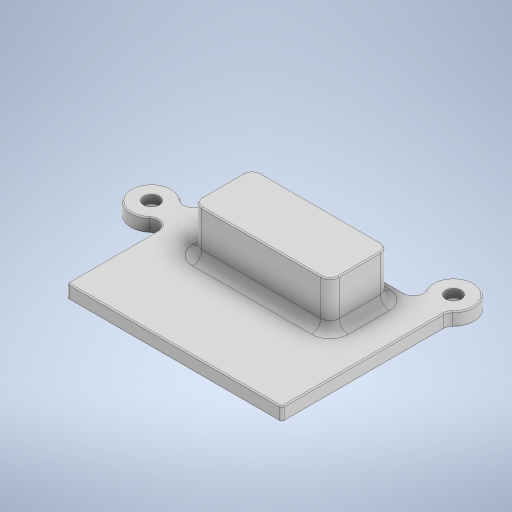
# Autodesk Inventor part: v2breadboardmount
Saved by Autodesk Inventor 2024.2 (Build 282272000, 272)
## iProperties
Created: 2024-01-13
Part Number: v2breadboardmount
Material: Generic
Document SubType Name: Modeling
Designer: Eric
Density: 1 g/cm^3
Appearance: Default
Author: Eric
Autodesk Inventor part; units mm, degrees
ref_plane "YZ Plane" through (0, 0, 0) normal (1, 0, 0) x (0, 1, 0)
ref_plane "XZ Plane" through (0, 0, 0) normal (0, 1, 0) x (-1, 0, 0)
ref_plane "XY Plane" through (0, 0, 0) normal (0, 0, 1) x (1, 0, 0)
sketch "Sketch1" plane through (0, 0, 0) normal (0, 1, 0) x (-1, 0, 0)
  line L0 (23.5, 17.5) -> (-23.5, 17.5)
  line L1 (-23.5, 17.5) -> (-23.5, -17.5)
  line L2 (-23.5, -17.5) -> (23.5, -17.5)
  line L3 (23.5, -17.5) -> (23.5, 17.5)
  line L4 (23.5, 17.5) -> (-23.5, -17.5) construction
  line L5 (-23.5, 17.5) -> (23.5, -17.5) construction
  circle A0 centre (-21, -22.5) radius 1.7
  circle A1 centre (-21, -22.5) radius 4.5
  line L6 (-23.5, -18.7583) -> (-23.5, -17.5)
  line L7 (-18.5, -17.5) -> (-18.5, -18.7583)
  circle A2 centre (29.8, -7.3) radius 1.7
  circle A3 centre (29.8, -7.3) radius 4.5
  line L8 (26.0583, -9.8) -> (23.5, -9.8)
  line L9 (23.5, -4.8) -> (26.0583, -4.8)
  point P0 (0, 0)
  point P1 (-16.8117, -24.1455)
  dimension "d0" = 47
  dimension "d1" = 35
  dimension "d3" = 3.4
  dimension "d4" = 5
  dimension "d5" = 9
  dimension "d17" = 2.5
  dimension "d18" = 5
  dimension "d19" = 50.8
  dimension "d20" = 5
  dimension "d21" = 2.5
  dimension "d22" = 15.2
  constraints: 20 end point, 5 point on circle, 4 centre point, 4 point on line, 3 parallel, 3 perpendicular, 2 coincident, 2 equal radius, 2 midpoint, 1 collinear, 1 horizontal, 1 vertical
  measures "d0" distance of L1.end L2.end
  measures "d1" distance between parallel lines of L0 L2
  measures "d3" diameter of A0
  measures "d4" distance from line of L2 A0.centre
  measures "d5" diameter of A1
  measures "d17" distance from line of L6 A0.centre
  measures "d18" distance between parallel lines of L6 L7
  measures "d19" horizontal distance of A0.centre A2.centre
  measures "d20" distance between parallel lines of L8 L9
  measures "d21" distance from line of L8 A2.centre
  measures "d22" vertical distance of A0.centre A2.centre
extrude "Extrusion1" add sketch "Sketch1" against normal blind 3
sketch "Sketch3" plane through (0, -3, 0) normal (0, 1, 0) x (1, 0, 0)
  circle A0 centre (-29.8, 7.3) radius 1.7 projected
  line L0 (-28.1546, 4.45) -> (-31.4454, 4.45)
  line L1 (-31.4454, 4.45) -> (-33.0909, 7.3)
  line L2 (-33.0909, 7.3) -> (-31.4454, 10.15)
  line L3 (-31.4454, 10.15) -> (-28.1546, 10.15)
  line L4 (-28.1546, 10.15) -> (-26.5091, 7.3)
  line L5 (-26.5091, 7.3) -> (-28.1546, 4.45)
  circle A1 centre (21, 22.5) radius 1.7 projected
  line L6 (21, 19.2091) -> (18.15, 20.8546)
  line L7 (18.15, 20.8546) -> (18.15, 24.1454)
  line L8 (18.15, 24.1454) -> (21, 25.7909)
  line L9 (21, 25.7909) -> (23.85, 24.1454)
  line L10 (23.85, 24.1454) -> (23.85, 20.8546)
  line L11 (23.85, 20.8546) -> (21, 19.2091)
  point P0 (0, 0)
  dimension "d23" = 5.7
  constraints: 24 end point, 2 coincident, 1 horizontal, 1 perpendicular, 1 vertical, 26 other
  measures "d23" distance between parallel lines of L10 L7
extrude "Extrusion3" cut sketch "Sketch3" along normal blind 1 contours A0 | L0 L1 L2 L3 L4 L5 | A1 | L6 L7 L8 L9 L10 L11
sketch "Sketch4" plane through (0, 0, 0) normal (0, 1, 0) x (1, 0, 0)
  line L0 (-15, 14.5) -> (15, 14.5)
  line L1 (15, 14.5) -> (15, 1.5)
  line L2 (15, 1.5) -> (-15, 1.5)
  line L3 (-15, 1.5) -> (-15, 14.5)
  line L4 (18.5, 17.5) -> (-23.5, 17.5) projected
  point P0 (0, 0)
  point P1 (0, 1.5)
  dimension "d26" = 30
  dimension "d27" = 13
  dimension "d28" = 3
  constraints: 8 end point, 2 parallel, 1 horizontal, 1 midpoint, 1 perpendicular, 1 vertical alignment
  measures "d26" distance between parallel lines of L1 L3
  measures "d27" distance between parallel lines of L2 L0
  measures "d28" distance between parallel lines of L4 L0
extrude "Extrusion4" add sketch "Sketch4" along normal blind 10
fillet "Fillet4" radius 2 15 edges at (-15, 5, -14.5) (-15, 5, -1.5) (15, 5, -14.5) (15, 5, -1.5) (0, 0, -14.5) (-15, 0, -8) (0, 0, -1.5) (15, 0, -8) (18.5, -1.5, -17.5) (18.5, -1.5, -18.7583) (23.5, -1.5, -18.7583) (-23.5, -1.5, -9.8) (-23.5, -1.5, -4.8) (-26.0583, -1.5, -4.8) (-26.0583, -1.5, -9.8)
fillet "Fillet5" radius 0.5 3 edges at (-23.5, -1.5, -17.5) (-23.5, -1.5, 17.5) (23.5, -1.5, 17.5)
fillet "Fillet6" radius 0.25 36 edges at (23.6603, 0, -18.594) (21.7305, 0, -26.9403) (16.9443, 0, -18.462) (-3.8823, 0, -17.5) (-23.3536, 0, -17.3536) (-23.5, 0, -14.5861) (-24.677, 0, -10.35) (-34.3, 0, -7.3) (-24.677, 0, -4.25) (-23.5, 0, 7.2861) (-23.3536, 0, 17.3536) (0, 0, 17.5) (23.3536, 0, 17.3536) (23.5, 0, -0.4048) (23.3536, -3, 17.3536) (0, -3, 17.5) (-23.3536, -3, 17.3536) (-23.5, -3, 7.2861) (-24.677, -3, -4.25) (-34.3, -3, -7.3) (-24.677, -3, -10.35) (-23.5, -3, -14.5861) (-23.3536, -3, -17.3536) (-3.8823, -3, -17.5) (16.9443, -3, -18.462) (21.7305, -3, -26.9403) (23.6603, -3, -18.594) (23.5, -3, -0.4048) (14.4142, 10, -13.9142) (0, 10, -14.5) (-14.4142, 10, -13.9142) (-15, 10, -8) (-14.4142, 10, -2.0858) (0, 10, -1.5) (14.4142, 10, -2.0858) (15, 10, -8)
sketch "Sketch5" plane through (0, -2, 0) normal (0, -1, 0) x (1, 0, 0)
  circle A0 centre (21, -22.5) radius 1.7 projected
  circle A1 centre (-29.8, -7.3) radius 1.7 projected
  point P0 (0, 0)
extrude "Extrusion5" add sketch "Sketch5" against normal blind 0.2
body "Solid1"
